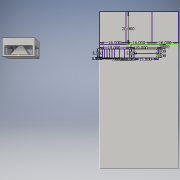
# Autodesk Inventor part: display version 3
Saved by Autodesk Inventor 2016 (Build 200138000, 138)
## iProperties
Created: 2017-10-10
Part Number: display version 3
Material: Generic
Document SubType Name: Modeling
Designer: student
Density: 1 g/cm^3
Appearance: Default
Author: student
Autodesk Inventor part; units mm, degrees
ref_plane "YZ Plane" through (0, 0, 0) normal (1, 0, 0) x (0, 1, 0)
ref_plane "XZ Plane" through (0, 0, 0) normal (0, 1, 0) x (-1, 0, 0)
sketch "Sketch1" plane through (0, 0, 0) normal (0, 0, 1) x (1, 0, 0)
  line L0 (-254, 12.7) -> (254, 12.7)
  line L1 (254, 12.7) -> (254, -12.7)
  line L2 (254, -12.7) -> (-254, -12.7)
  line L3 (-254, -12.7) -> (-254, 12.7)
  point P0 (0, 0)
  point P1 (0, -12.7)
  point P2 (254, 0)
  dimension "d0" = 25.4
  dimension "d1" = 508
  constraints: 8 end point, 2 midpoint, 2 parallel, 1 horizontal, 1 horizontal alignment, 1 perpendicular, 1 vertical alignment
  measures "d0" distance of L0.end L1.end
  measures "d1" distance of L0.start L0.end
extrude "Extrusion1" add sketch "Sketch1" along normal blind 406.4
sketch "Sketch2" plane through (-254, 12.7, 0) normal (0, 1, 0) x (1, 0, 0)
  line L0 (403.225, -53.975) -> (403.225, -352.425)
  line L1 (403.225, -352.425) -> (104.775, -352.425)
  line L2 (104.775, -352.425) -> (104.775, -53.975)
  line L3 (104.775, -53.975) -> (403.225, -53.975)
  line L4 (0, 0) -> (0, -406.4) projected
  line L5 (0, 0) -> (508, 0) projected
  point P0 (254, 0)
  point P1 (254, -203.2)
  point P2 (0, -203.2)
  point P3 (254, 0)
  dimension "d4" = 298.45
  constraints: 8 end point, 2 midpoint, 1 horizontal alignment, 1 vertical alignment, 9 other
  measures "d4" distance of L2.end L0.start
ref_plane "Work Plane1" through (-254, 177.8, 0) normal (0, 1, 0) x (1, 0, 0)
sketch "Sketch3" plane through (-254, 177.8, 0) normal (0, 1, 0) x (1, 0, 0)
  line L0 (285.75, -171.45) -> (285.75, -234.95)
  line L1 (285.75, -234.95) -> (222.25, -234.95)
  line L2 (222.25, -234.95) -> (222.25, -171.45)
  line L3 (222.25, -171.45) -> (285.75, -171.45)
  line L4 (0, 0) -> (0, -406.4) projected
  point P0 (254, 0)
  point P1 (254, -203.2)
  point P2 (0, -203.2)
  dimension "d6" = 63.5
  constraints: 8 end point, 1 horizontal alignment, 1 midpoint, 1 vertical alignment, 9 other
  measures "d6" distance of L2.end L0.start
loft "Loft1" add profiles "Sketch3", "Sketch2"
sketch "Sketch4" plane through (-31.75, 177.8, 171.45) normal (0, 1, 0) x (1, 0, 0)
  line L0 (-173.99, 137.16) -> (237.49, 137.16)
  line L1 (237.49, 137.16) -> (237.49, -200.66)
  line L2 (237.49, -200.66) -> (-173.99, -200.66)
  line L3 (-173.99, -200.66) -> (-173.99, 137.16)
  line L4 (285.75, 171.45) -> (285.75, -234.95) projected
  point P0 (31.75, 171.45)
  point P1 (31.75, 137.16)
  point P2 (237.49, -31.75)
  point P3 (285.75, -31.75)
  dimension "d11" = 411.48
  dimension "d12" = 337.82
  constraints: 8 end point, 3 midpoint, 2 parallel, 1 horizontal, 1 horizontal alignment, 1 perpendicular, 1 vertical alignment
  measures "d11" distance of L0.start L0.end
  measures "d12" distance of L0.end L1.end
extrude "Extrusion2" add sketch "Sketch4" along normal blind 65.024
sketch "Sketch5" plane through (-205.74, 177.8, 372.11) normal (0, 0, 1) x (1, 0, 0)
  line L0 (0, 0) -> (0, 23.876)
  line L1 (0, 0) -> (0, 65.024) projected
  line L2 (102.87, 65.024) -> (308.61, 65.024)
  line L3 (0, 23.876) -> (102.87, 65.024)
  line L4 (0, 65.024) -> (411.48, 65.024) projected
  line L5 (0, 65.024) -> (102.87, 65.024)
  line L6 (0, 65.024) -> (0, 23.876)
  line L7 (308.61, 65.024) -> (411.48, 23.876)
  line L8 (411.48, 23.876) -> (411.48, 65.024)
  line L9 (411.48, 65.024) -> (308.61, 65.024)
  point P0 (205.74, -177.8)
  point P1 (205.74, 65.024)
  point P2 (205.74, 0)
  dimension "d15" = 23.876
  dimension "d16" = 205.74
  constraints: 16 end point, 2 collinear, 1 midpoint, 1 perpendicular, 1 point on line, 1 vertical, 1 vertical alignment
  measures "d15" distance of L0.start L0.end
  measures "d16" distance of L2.start L2.end
extrude "Extrusion3" cut sketch "Sketch5" against normal blind 390.5885
sketch "Sketch6" plane through (-254, 12.7, 0) normal (0, 1, 0) x (1, 0, 0)
  line L0 (0, 0) -> (76.2, 0)
  line L1 (76.2, 0) -> (76.2, -76.2)
  line L2 (76.2, -76.2) -> (0, -76.2)
  line L3 (0, -76.2) -> (0, 0)
  line L4 (0, -406.4) -> (38.1, -406.4)
  line L5 (38.1, -406.4) -> (38.1, -368.3)
  line L6 (38.1, -368.3) -> (0, -368.3)
  line L7 (0, -368.3) -> (0, -406.4)
  line L8 (508, 0) -> (469.9, 0)
  line L9 (469.9, 0) -> (469.9, -38.1)
  line L10 (469.9, -38.1) -> (508, -38.1)
  line L11 (508, -38.1) -> (508, 0)
  line L12 (508, -406.4) -> (469.9, -406.4)
  line L13 (508, -368.3) -> (508, -406.4)
  line L14 (469.9, -368.3) -> (508, -368.3)
  line L15 (469.9, -406.4) -> (469.9, -368.3)
  point P0 (254, 0)
  point P1 (38.1, -38.1)
  point P2 (38.1, 0)
  dimension "d19" = 76.2
  constraints: 32 end point, 1 horizontal, 1 horizontal alignment, 1 midpoint, 1 vertical, 9 other
  measures "d19" distance of L1.end L2.end
extrude "Extrusion4" add sketch "Sketch6" along normal blind 139.7
sketch "Sketch7" plane through (-254, 152.4, 0) normal (0, 1, 0) x (1, 0, 0)
  line L0 (469.9, -406.4) -> (508, -406.4)
  line L1 (0, 0) -> (508, 0)
  line L2 (508, 0) -> (508, -406.4)
  line L3 (508, -406.4) -> (0, -406.4)
  line L4 (0, -406.4) -> (0, 0)
  line L5 (69.85, -31.75) -> (438.15, -31.75)
  line L6 (438.15, -31.75) -> (438.15, -374.65)
  line L7 (438.15, -374.65) -> (69.85, -374.65)
  line L8 (69.85, -374.65) -> (69.85, -31.75)
  line L9 (469.9, -368.3) -> (469.9, -406.4)
  line L10 (38.1, -406.4) -> (38.1, -368.3)
  line L11 (38.1, -38.1) -> (38.1, 0)
  line L12 (469.9, 0) -> (469.9, -38.1)
  point P0 (254, 0)
  point P1 (254, 0)
  dimension "d22" = 31.75
  dimension "d23" = 31.75
  dimension "d24" = 31.75
  dimension "d25" = 31.75
  dimension "d26" = 31.75
  dimension "d27" = 31.75
  constraints: 26 end point, 4 parallel, 2 horizontal, 2 perpendicular
  measures "d22" distance from line of L9 L6.end
  measures "d23" distance between parallel lines of L3 L7
  measures "d24" distance between parallel lines of L10 L8
  measures "d25" distance between parallel lines of L11 L8
  measures "d26" distance between parallel lines of L12 L6
  measures "d27" distance between parallel lines of L1 L5
extrude "Extrusion5" add sketch "Sketch7" along normal blind 25.4
sketch "Sketch8" plane through (-254, 177.8, 0) normal (0, 1, 0) x (1, 0, 0)
  line L0 (0, 0) -> (508, 0)
  line L1 (508, 0) -> (508, -406.4)
  line L2 (508, -406.4) -> (0, -406.4)
  line L3 (0, -406.4) -> (0, 0)
  line L4 (25.4, -25.4) -> (482.6, -25.4)
  line L5 (482.6, -25.4) -> (482.6, -381)
  line L6 (482.6, -381) -> (25.4, -381)
  line L7 (25.4, -381) -> (25.4, -25.4)
  line L8 (304.8, 0) -> (304.8, -25.4)
  line L9 (304.8, -25.4) -> (203.2, -25.4)
  line L10 (203.2, -25.4) -> (203.2, 0)
  point P0 (254, 0)
  point P1 (254, 0)
  dimension "d30" = 25.4
  dimension "d31" = 25.4
  dimension "d32" = 25.4
  dimension "d33" = 25.4
  constraints: 22 end point, 5 parallel, 3 point on line, 2 horizontal, 2 perpendicular
  measures "d30" distance between parallel lines of L0 L4
  measures "d31" distance between parallel lines of L3 L7
  measures "d32" distance between parallel lines of L1 L5
  measures "d33" distance between parallel lines of L2 L6
extrude "Extrusion6" add sketch "Sketch8" along normal blind 71.12 contours L0 L10 L4 L7 L6 L5 L8 L1 L2 L3
sketch "Sketch9" plane through (0, 0, 406.4) normal (0, 0, 1) x (1, 0, 0)
  line L0 (-254, 248.92) -> (254, 248.92) projected
  line L1 (-254, 248.92) -> (254, 248.92)
  line L2 (254, 248.92) -> (254, 274.32)
  line L3 (254, 274.32) -> (-254, 274.32)
  line L4 (-254, 274.32) -> (-254, 248.92)
  line L5 (254, -12.7) -> (254, 248.92) projected
  point P0 (0, 0)
  point P1 (254, 261.62)
  point P2 (254, 118.11)
  dimension "d36" = 25.4
  constraints: 8 end point, 2 midpoint, 2 parallel, 2 vertical alignment, 1 horizontal, 1 perpendicular
  measures "d36" distance of L1.end L2.end
extrude "Extrusion7" add sketch "Sketch9" against normal blind 406.4
sketch "Sketch10" plane through (0, 0, 406.4) normal (0, 0, 1) x (1, 0, 0)
  line L0 (1262.5907, 679.0542) -> (2481.7907, 679.0542)
  line L1 (2481.7907, 679.0542) -> (2481.7907, -1759.3458)
  line L2 (2481.7907, -1759.3458) -> (1262.5907, -1759.3458)
  line L3 (1262.5907, -1759.3458) -> (1262.5907, 679.0542)
  point P0 (0, 0)
  dimension "d39" = 1219.2
  dimension "d40" = 2438.4
  constraints: 8 end point, 2 parallel, 1 horizontal, 1 perpendicular
  measures "d39" distance of L0.start L0.end
  measures "d40" distance of L0.end L1.end
extrude "Extrusion8" add sketch "Sketch10" along normal blind 19.05
sketch "Sketch11" plane through (0, 0, 425.45) normal (0, 0, 1) x (1, 0, 0)
  line L0 (1262.5907, 679.0542) -> (1262.5907, -1759.3458) projected
  line L1 (1262.5907, 679.0542) -> (1668.9907, 679.0542)
  line L2 (1668.9907, 679.0542) -> (1668.9907, 171.0542)
  line L3 (1668.9907, 171.0542) -> (1262.5907, 171.0542)
  line L4 (1262.5907, 171.0542) -> (1262.5907, 679.0542)
  line L5 (1668.9907, 679.0542) -> (2075.3907, 679.0542)
  line L6 (2075.3907, 679.0542) -> (2075.3907, 171.0542)
  line L7 (2075.3907, 171.0542) -> (1668.9907, 171.0542)
  line L8 (1668.9907, 171.0542) -> (1668.9907, 679.0542)
  line L9 (2075.3907, 679.0542) -> (2481.7907, 679.0542)
  line L10 (2481.7907, 679.0542) -> (2481.7907, 171.0542)
  line L11 (2481.7907, 171.0542) -> (2075.3907, 171.0542)
  line L12 (2075.3907, 171.0542) -> (2075.3907, 679.0542)
  line L13 (1262.5907, 171.0542) -> (1745.1907, 171.0542)
  line L14 (1745.1907, 171.0542) -> (1745.1907, 99.9342)
  line L15 (1745.1907, 99.9342) -> (1262.5907, 99.9342)
  line L16 (1262.5907, 99.9342) -> (1262.5907, 171.0542)
  line L17 (1745.1907, 99.9342) -> (2227.7907, 99.9342)
  line L18 (2227.7907, 99.9342) -> (2227.7907, 171.0542)
  line L19 (2227.7907, 171.0542) -> (1745.1907, 171.0542)
  line L20 (1745.1907, 171.0542) -> (1745.1907, 99.9342)
  line L21 (2298.9107, 171.0542) -> (2227.7907, 171.0542)
  line L22 (2298.9107, 171.0542) -> (2370.0307, 171.0542)
  line L23 (1262.5907, 99.9342) -> (1300.6907, 99.9342)
  line L24 (1300.6907, 99.9342) -> (1300.6907, -39.7658)
  line L25 (1300.6907, -39.7658) -> (1262.5907, -39.7658)
  line L26 (1262.5907, -39.7658) -> (1262.5907, 99.9342)
  line L27 (1300.6907, 99.9342) -> (1338.7907, 99.9342)
  line L28 (1338.7907, 99.9342) -> (1338.7907, -39.7658)
  line L29 (1338.7907, -39.7658) -> (1300.6907, -39.7658)
  line L30 (1300.6907, -39.7658) -> (1300.6907, 99.9342)
  line L31 (1338.7907, 99.9342) -> (1376.8907, 99.9342)
  line L32 (1376.8907, 99.9342) -> (1376.8907, -39.7658)
  line L33 (1376.8907, -39.7658) -> (1338.7907, -39.7658)
  line L34 (1338.7907, -39.7658) -> (1338.7907, 99.9342)
  line L35 (1376.8907, 99.9342) -> (1414.9907, 99.9342)
  line L36 (1414.9907, 99.9342) -> (1414.9907, -39.7658)
  line L37 (1414.9907, -39.7658) -> (1376.8907, -39.7658)
  line L38 (1376.8907, -39.7658) -> (1376.8907, 99.9342)
  line L39 (1414.9907, 99.9342) -> (1453.0907, 99.9342)
  line L40 (1453.0907, 99.9342) -> (1453.0907, -39.7658)
  line L41 (1453.0907, -39.7658) -> (1414.9907, -39.7658)
  line L42 (1414.9907, -39.7658) -> (1414.9907, 99.9342)
  line L43 (1453.0907, 99.9342) -> (1491.1907, 99.9342)
  line L44 (1491.1907, 99.9342) -> (1491.1907, -39.7658)
  line L45 (1491.1907, -39.7658) -> (1453.0907, -39.7658)
  line L46 (1453.0907, -39.7658) -> (1453.0907, 99.9342)
  line L47 (1491.1907, 99.9342) -> (1567.3907, 99.9342)
  line L48 (1567.3907, 99.9342) -> (1567.3907, -39.7658)
  line L49 (1567.3907, -39.7658) -> (1491.1907, -39.7658)
  line L50 (1491.1907, -39.7658) -> (1491.1907, 99.9342)
  line L51 (1567.3907, 99.9342) -> (1643.5907, 99.9342)
  line L52 (1643.5907, 99.9342) -> (1643.5907, -39.7658)
  line L53 (1643.5907, -39.7658) -> (1567.3907, -39.7658)
  line L54 (1567.3907, -39.7658) -> (1567.3907, 99.9342)
  line L55 (1643.5907, 99.9342) -> (1719.7907, 99.9342)
  line L56 (1719.7907, 99.9342) -> (1719.7907, -39.7658)
  line L57 (1719.7907, -39.7658) -> (1643.5907, -39.7658)
  line L58 (1643.5907, -39.7658) -> (1643.5907, 99.9342)
  line L59 (1719.7907, 99.9342) -> (1795.9907, 99.9342)
  line L60 (1795.9907, 99.9342) -> (1795.9907, -39.7658)
  line L61 (1795.9907, -39.7658) -> (1719.7907, -39.7658)
  line L62 (1719.7907, -39.7658) -> (1719.7907, 99.9342)
  line L63 (1795.9907, 99.9342) -> (2176.9907, 99.9342)
  line L64 (2176.9907, 99.9342) -> (2176.9907, 28.8142)
  line L65 (2176.9907, 28.8142) -> (1795.9907, 28.8142)
  line L66 (1795.9907, 28.8142) -> (1795.9907, 99.9342)
  line L67 (1795.9907, 28.8142) -> (2176.9907, 28.8142)
  line L68 (2176.9907, 28.8142) -> (2176.9907, -42.3058)
  line L69 (2176.9907, -42.3058) -> (1795.9907, -42.3058)
  line L70 (1795.9907, -42.3058) -> (1795.9907, 28.8142)
  point P0 (0, 0)
  dimension "d43" = 508
  dimension "d44" = 406.4
  dimension "d45" = 406.4
  dimension "d46" = 406.4
  dimension "d47" = 71.12
  dimension "d48" = 482.6
  dimension "d49" = 482.6
  dimension "d53" = 139.7
  dimension "d54" = 38.1
  dimension "d55" = 38.1
  dimension "d56" = 38.1
  dimension "d57" = 38.1
  dimension "d58" = 38.1
  dimension "d59" = 38.1
  dimension "d60" = 76.2
  dimension "d61" = 76.2
  dimension "d62" = 76.2
  dimension "d63" = 76.2
  dimension "d64" = 139.7
  dimension "d65" = 381
  dimension "d66" = 71.12
  dimension "d67" = 71.12
  constraints: 140 end point, 34 parallel, 19 horizontal, 17 perpendicular, 7 point on line
  measures "d43" distance of L1.end L2.end
  measures "d44" distance of L2.end L3.end
  measures "d45" distance of L6.end L7.end
  measures "d46" distance of L10.end L11.end
  measures "d47" distance of L13.end L14.end
  measures "d48" distance of L14.end L15.end
  measures "d49" distance of L14.end L17.end
  measures "d53" distance of L23.end L24.end
  measures "d54" distance of L24.end L25.end
  measures "d55" distance of L28.end L29.end
  measures "d56" distance of L32.end L33.end
  measures "d57" distance of L36.end L37.end
  measures "d58" distance of L40.end L41.end
  measures "d59" distance of L44.end L45.end
  measures "d60" distance of L48.end L49.end
  measures "d61" distance of L52.end L53.end
  measures "d62" distance of L56.end L57.end
  measures "d63" distance of L60.end L61.end
  measures "d64" distance of L59.end L60.end
  measures "d65" distance of L64.end L65.end
  measures "d66" distance of L63.end L64.end
  measures "d67" distance of L67.end L68.end
body "Solid1"
